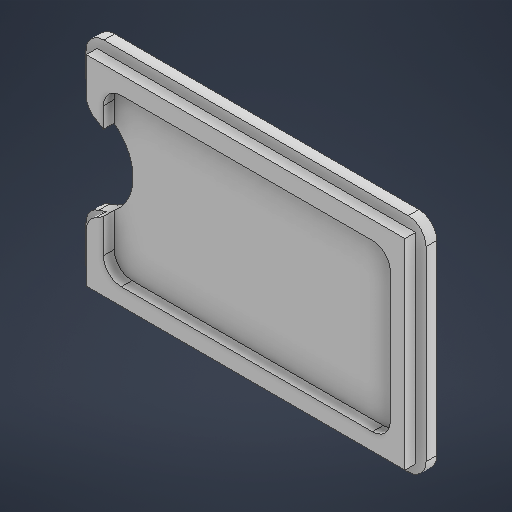
# Autodesk Inventor part: top
Saved by Autodesk Inventor 2026.1 (Build 301233020, 233B)
## iProperties
Created: 2025-11-06
Part Number: top
Material: Generisch
Document SubType Name: Modeling
Designer: sarae
Density: 1 g/cm^3
Appearance: Vorgabe
Author: sarae
Autodesk Inventor part; units mm, degrees
ref_plane "YZ Plane" through (0, 0, 0) normal (1, 0, 0) x (0, 1, 0)
ref_plane "XZ Plane" through (0, 0, 0) normal (0, 1, 0) x (-1, 0, 0)
ref_plane "XY Plane" through (0, 0, 0) normal (0, 0, 1) x (1, 0, 0)
sketch "Skizze1" plane through (0, 0, 0) normal (0, 1, 0) x (-1, 0, 0)
  line L0 (-53.2068, 33.801) -> (41.7932, 33.801)
  line L1 (41.7932, 33.801) -> (41.7932, -28.199)
  line L2 (41.7932, -28.199) -> (-53.2068, -28.199)
  line L3 (-53.2068, -28.199) -> (-53.2068, 33.801)
  line L4 (-50.2068, 30.801) -> (38.7932, 30.801)
  line L5 (38.7932, 30.801) -> (38.7932, -25.199)
  line L6 (38.7932, -25.199) -> (-50.2068, -25.199)
  line L7 (-50.2068, -25.199) -> (-50.2068, 30.801)
  point P0 (0, 0)
  point P1 (-48.7827, 30.712)
  dimension "d0" = 95
  dimension "d1" = 62
  dimension "d2" = 89
  dimension "d3" = 56
  dimension "d4" = 3
  dimension "d5" = 3
  constraints: 16 end point, 4 parallel, 2 horizontal, 2 perpendicular
  measures "d0" distance of L1.end L2.end
  measures "d1" distance of L0.end L1.end
  measures "d2" distance of L5.end L6.end
  measures "d3" distance of L4.end L5.end
  measures "d4" distance between parallel lines of L0 L4
  measures "d5" distance between parallel lines of L7 L3
extrude "Extrusion1" add sketch "Skizze1" along normal blind 3 contours L0 L1 L2 L3 | L4 L5 L6 L7
fillet "Rundung1" radius 5 4 edges at (-41.7932, 1.5, -28.199) (53.2068, 1.5, -28.199) (-41.7932, 1.5, 33.801) (53.2068, 1.5, 33.801)
sketch "Skizze2" plane through (0, 0, 0) normal (0, -1, 0) x (1, 0, 0)
  line L0 (-41.6836, 33.8201) -> (53.3164, 33.8201)
  line L1 (53.3164, 33.8201) -> (53.3164, -28.1799)
  line L2 (53.3164, -28.1799) -> (-41.6836, -28.1799)
  line L3 (-41.6836, -28.1799) -> (-41.6836, 33.8201)
  line L4 (-38.6836, 30.8201) -> (50.3164, 30.8201)
  line L5 (50.3164, 30.8201) -> (50.3164, -25.1799)
  line L6 (50.3164, -25.1799) -> (-38.6836, -25.1799)
  line L7 (-38.6836, -25.1799) -> (-38.6836, 30.8201)
  line L8 (46.2352, 25.8167) -> (-33.9228, 25.8167)
  line L9 (-33.9228, 25.8167) -> (-33.9228, -20.451)
  line L10 (-33.9228, -20.451) -> (46.2352, -20.451)
  line L11 (46.2352, -20.451) -> (46.2352, 25.8167)
  point P0 (0, 0)
  point P1 (-89.6071, 35.7543)
  dimension "d9" = 95
  dimension "d10" = 62
  dimension "d11" = 89
  dimension "d12" = 56
  dimension "d13" = 3
  dimension "d14" = 3
  constraints: 24 end point, 6 parallel, 3 horizontal, 3 perpendicular
  measures "d9" distance of L1.end L2.end
  measures "d10" distance of L0.end L1.end
  measures "d11" distance of L5.end L6.end
  measures "d12" distance of L4.end L5.end
  measures "d13" distance between parallel lines of L0 L4
  measures "d14" distance between parallel lines of L7 L3
extrude "Extrusion2" add sketch "Skizze2" along normal blind 3 contours L4 L5 L6 L7
sketch "Skizze3" plane through (0, 3, 0) normal (0, 1, 0) x (1, 0, 0)
  line L0 (-41.7932, 23.199) -> (-41.7932, -28.801) projected
  circle A0 centre (-41.7932, -4.5874) radius 13.1555
  point P0 (0, 0)
  point P1 (-41.7932, 8.5681)
  point P2 (-41.7932, -17.7429)
  constraints: 1 centre point, 1 point on line
extrude "Extrusion3" cut sketch "Skizze3" against normal blind 6 contours A0 L0 picked at (-38.9148, -0.5266)
fillet "Rundung2" radius 5 4 edges at (-41.7932, 1.5, 17.7429) (-41.7932, 1.5, -8.5681) (-38.6836, -1.5, -8.1953) (-38.6836, -1.5, 17.3701)
fillet "Rundung3" radius 5 4 edges at (46.2352, -1.5, 25.8167) (46.2352, -1.5, -20.451) (-33.9228, -1.5, -20.451) (-33.9228, -1.5, 25.8167)
